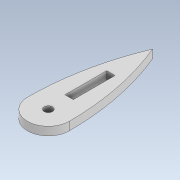
# Autodesk Inventor part: aileron_arriere
Saved by Autodesk Inventor 2020 (Build 240168000, 168)
## iProperties
Created: 2020-09-10
Part Number: aileron_arriere
Material: Generic
Document SubType Name: Modeling
Designer: Admin
Density: 1 g/cm^3
Appearance: Default
Author: Admin
Autodesk Inventor part; units mm, degrees
ref_plane "YZ Plane" through (0, 0, 0) normal (1, 0, 0) x (0, 1, 0)
ref_plane "XZ Plane" through (0, 0, 0) normal (0, 1, 0) x (-1, 0, 0)
ref_plane "XY Plane" through (0, 0, 0) normal (0, 0, 1) x (1, 0, 0)
sketch "Sketch1" plane through (0, 0, 0) normal (0, 1, 0) x (-1, 0, 0)
  arc A0 (5, 0) -> (-5, 0) centre (0, 0) ccw
  arc A1 (0, -25) -> (5, 0) centre (-60, 0) ccw
  arc A2 (-5, 0) -> (0, -25) centre (60, 0) ccw
  circle A3 centre (0, 0) radius 1
  line L0 (1, -5) -> (-1, -5)
  line L1 (-1, -5) -> (-1, -15)
  line L2 (-1, -15) -> (1, -15)
  line L3 (1, -15) -> (1, -5)
  dimension "d0" = 5
  dimension "d1" = 0
  dimension "d2" = 0
  dimension "d3" = 0
  dimension "d4" = 0
  dimension "d5" = 0
  dimension "d6" = 25
  dimension "d7" = 2
  dimension "d10" = 10
  dimension "d11" = 2
  dimension "d12" = 1
  dimension "d13" = 5
  constraints: 8 end point, 6 point on circle, 4 centre point, 2 coincident, 2 parallel, 1 horizontal, 1 perpendicular
  measures "d0" radius of A0
  measures "d1" vertical distance of point (0, 0) A0.start
  measures "d2" vertical distance of point (0, 0) A0.end
  measures "d3" vertical distance of point (0, 0) A2.centre
  measures "d4" vertical distance of point (0, 0) A1.centre
  measures "d5" horizontal distance of point (0, 0) A1.start
  measures "d6" distance of point (0, 0) A1.start
  measures "d7" diameter of A3
  measures "d10" distance of L2.end L0.start
  measures "d11" distance of L0.start L0.end
  measures "d12" distance from line of point (0, 0) L3
  measures "d13" distance from line of L0 point (0, 0)
extrude "Extrusion2" add sketch "Sketch1" along normal blind 2
body "Solid2"
